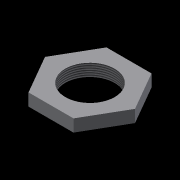
# Autodesk Inventor part: 3d_LM-Welding_Tooling -  Micrometer Nut
Saved by Autodesk Inventor 2018.3 (Build 223284000, 284)
## iProperties
Created: 2026-01-29
Part Number: 3d_LM-Welding_Tooling -  Micrometer Nut
Material: Genérico
Document SubType Name: Modeling
Designer: aca6
Density: 1 g/cm^3
Appearance: Valor por defecto
Author: aca6
Autodesk Inventor part; units mm, degrees
ref_plane "YZ Plane" through (0, 0, 0) normal (1, 0, 0) x (0, 1, 0)
ref_plane "XZ Plane" through (0, 0, 0) normal (0, 1, 0) x (-1, 0, 0)
ref_plane "XY Plane" through (0, 0, 0) normal (0, 0, 1) x (1, 0, 0)
sketch "Sketch1" plane through (0, 0, 0) normal (0, 0, 1) x (1, 0, 0)
  line L0 (10.9697, 0) -> (5.4848, -9.5)
  line L1 (5.4848, -9.5) -> (-5.4848, -9.5)
  line L2 (-5.4848, -9.5) -> (-10.9697, 0)
  line L3 (-10.9697, 0) -> (-5.4848, 9.5)
  line L4 (-5.4848, 9.5) -> (5.4848, 9.5)
  line L5 (5.4848, 9.5) -> (10.9697, 0)
  circle A0 centre (0, 0) radius 6
  dimension "d0" = 12
  dimension "d1" = 19
  constraints: 12 end point, 2 coincident, 1 centre point, 13 other
  measures "d0" diameter of A0
  measures "d1" distance between parallel lines of L0 L3
extrude "Extrusion1" add sketch "Sketch1" along normal blind 3
thread "Thread1" size "M12x0.5" class "6H" standard "ISO Metric profile" full length
body "Solid1"
